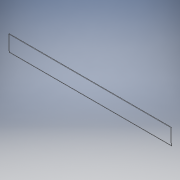
# Autodesk Inventor part: element_2
Saved by Autodesk Inventor 2018.1 (Build 221171000, 171)
## iProperties
Created: 2017-10-22
Part Number: element_2
Material: CFRP
Document SubType Name: Modeling
Designer: ku_sk
Density: 1.43 g/cm^3
Appearance: カーボンファイバー
Mass: 645.479 g
Surface Area: 1958.96 cm^2
Volume: 451.384 cm^3
Author: ku_sk
Autodesk Inventor part; units mm, degrees
ref_plane "YZ Plane" through (0, 0, 0) normal (1, 0, 0) x (0, 1, 0)
ref_plane "XZ Plane" through (0, 0, 0) normal (0, 1, 0) x (-1, 0, 0)
ref_plane "XY Plane" through (0, 0, 0) normal (0, 0, 1) x (1, 0, 0)
sketch "スケッチ1" plane through (0, 0, 0) normal (1, 0, 0) x (0, 1, 0)
  line L0 (0, 70) -> (0, -70)
  arc A0 (0, 70) -> (0, -70) centre (636.1604, 0) ccw
  arc A1 (0, 70) -> (0, -70) centre (250.3997, 0) ccw
  line L1 (-138.7525, 0) -> (765.3125, 0) projected
  point P0 (0, 0)
  point P1 (0, 0)
  dimension "d2" = 140
  dimension "d3" = 640
  dimension "d4" = 260
  constraints: 4 point on circle, 2 centre point, 2 end point, 2 midpoint, 1 point on line, 1 vertical
  measures "d2" distance of L0.start L0.end
  measures "d3" radius of A0
  measures "d4" radius of A1
extrude "押し出し1" add sketch "スケッチ1" along normal mid plane 970 contours A0 L1 A1 | A0 A1 L1
fillet "フィレット1" radius 2 1 edges at (0, 0, 70)
fillet "フィレット2" radius 1 1 edges at (0, 0, -70)
